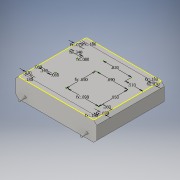
# Autodesk Inventor part: Chassis
Saved by Autodesk Inventor 2016 (Build 200138000, 138)
## iProperties
Created: 2015-09-02
Part Number: Chassis
Material: Generic
Document SubType Name: Modeling
Designer: lachesis
Density: 1 g/cm^3
Appearance: Default
Author: lachesis
Autodesk Inventor part; units mm, degrees
ref_plane "YZ Plane" through (0, 0, 0) normal (1, 0, 0) x (0, 1, 0)
ref_plane "XZ Plane" through (0, 0, 0) normal (0, 1, 0) x (-1, 0, 0)
ref_plane "XY Plane" through (0, 0, 0) normal (0, 0, 1) x (1, 0, 0)
sketch "Sketch1" plane through (0, 0, 0) normal (0, 0, 1) x (1, 0, 0)
  line L0 (-27.3831, 7.112) -> (27.3831, 7.112)
  line L1 (29.718, 4.7771) -> (29.718, -4.7771)
  line L2 (27.3831, -7.112) -> (-27.3831, -7.112)
  line L3 (-29.718, -4.7771) -> (-29.718, 4.7771)
  line L4 (-27.3831, 7.112) -> (-29.718, 4.7771)
  line L5 (-29.718, -4.7771) -> (-27.3831, -7.112)
  line L6 (27.3831, 7.112) -> (29.718, 4.7771)
  line L7 (29.718, -4.7771) -> (27.3831, -7.112)
  point P0 (0, 0)
  point P1 (-29.718, 7.112)
  point P2 (29.718, -7.112)
  point P3 (29.718, 7.112)
  point P4 (-29.718, -7.112)
  point P5 (29.718, 0)
  point P6 (0, 7.112)
  dimension "d0" = 59.436
  dimension "d1" = 14.224
  dimension "d4" = 3.302
  dimension "d5" = 135
  dimension "d7" = 45
  dimension "d8" = 3.302
  dimension "d10" = 45
  dimension "d11" = 3.302
  dimension "d13" = 45
  dimension "d14" = 3.302
  constraints: 16 end point, 8 point on line, 2 midpoint, 2 parallel, 1 horizontal, 1 horizontal alignment, 1 perpendicular, 1 vertical alignment
  measures "d0" distance between parallel lines of L1 L3
  measures "d1" distance between parallel lines of L0 L2
  measures "d4" distance of L0.start L3.end
  measures "d5" angle of L3 L4
  measures "d7" angle of L3 L5
  measures "d8" distance of L3.start L2.end
  measures "d10" angle of L0 L6
  measures "d11" distance of L0.end L1.start
  measures "d13" angle of L1 L7
  measures "d14" distance of L1.end L2.start
extrude "Extrusion1" add sketch "Sketch1" along normal blind 49.276
sketch "Sketch2" plane through (0, 0, 49.276) normal (0, 0, 1) x (1, 0, 0)
  circle A0 centre (-22.606, -3.556) radius 0.762
  line L0 (-27.3831, -7.112) -> (27.3831, -7.112) projected
  circle A1 centre (22.606, -3.556) radius 0.762
  line L1 (-29.718, 4.7771) -> (-29.718, -4.7771) projected
  line L2 (29.718, -4.7771) -> (29.718, 4.7771) projected
  point P0 (0, 0)
  dimension "d17" = 3.556
  dimension "d18" = 3.556
  dimension "d19" = 1.524
  dimension "d20" = 1.524
  dimension "d21" = 7.112
  dimension "d22" = 7.112
  constraints: 2 centre point
  measures "d17" distance from line of L0 A0.centre
  measures "d18" distance from line of L0 A1.centre
  measures "d19" diameter of A0
  measures "d20" diameter of A1
  measures "d21" distance from line of L1 A0.centre
  measures "d22" distance from line of L2 A1.centre
extrude "Extrusion2" add sketch "Sketch2" along normal blind 4.318
sketch "Sketch3" plane through (0, 0, 0) normal (0, 0, -1) x (-1, 0, 0)
  circle A0 centre (22.606, -3.556) radius 0.762 projected
  circle A1 centre (-22.606, -3.556) radius 0.762 projected
  circle A2 centre (-22.606, -3.556) radius 0.762
  circle A3 centre (22.606, -3.556) radius 0.762
  point P0 (0, 0)
  constraints: 2 centre point, 2 coincident, 2 concentric
extrude "Extrusion3" add sketch "Sketch3" along normal blind 4.318
sketch "Sketch4" plane through (-27.3831, 7.112, 0) normal (0, 1, 0) x (1, 0, 0)
  line L0 (0, 0) -> (0, -49.276) projected
  line L1 (54.7663, 0) -> (54.7663, -49.276) projected
  line L2 (0, -3.302) -> (54.7663, -3.302)
  line L3 (54.7663, -3.302) -> (54.7663, -45.974)
  line L4 (54.7663, -45.974) -> (0, -45.974)
  line L5 (0, -45.974) -> (0, -3.302)
  point P0 (27.3831, 0)
  dimension "d30" = 42.672
  dimension "d31" = 3.302
  constraints: 8 end point, 2 parallel, 2 point on line, 1 horizontal, 1 perpendicular
  measures "d30" distance between parallel lines of L4 L2
  measures "d31" distance from line of point (27.383, 0) L2
extrude "Extrusion4" cut sketch "Sketch4" against normal blind 11.8872
sketch "Sketch5" plane through (-27.3831, 7.112, 0) normal (0, 1, 0) x (1, 0, 0)
  line L0 (0, 0) -> (-2.3349, 0) projected
  line L1 (54.7663, -3.302) -> (54.7663, -45.974) projected
  line L2 (0, 0) -> (54.7663, 0)
  line L3 (54.7663, 0) -> (54.7663, -45.974)
  line L4 (54.7663, -45.974) -> (0, -45.974)
  line L5 (0, -45.974) -> (0, 0)
  point P0 (27.3831, 0)
  constraints: 8 end point, 2 parallel, 1 horizontal, 1 perpendicular
extrude "Extrusion5" add sketch "Sketch5" against normal blind 0.8128 separate body
sketch "Sketch6" plane through (-27.3831, 7.112, 0) normal (0, 1, 0) x (1, 0, 0)
  line L0 (0, -3.302) -> (0, -45.974) projected
  line L1 (54.7663, -3.302) -> (54.7663, -45.974) projected
  line L2 (54.7663, -49.276) -> (0, -49.276) projected
  line L3 (54.7663, 0) -> (0, 0) projected
  line L4 (0, 0) -> (0, -3.302) projected
  line L5 (0, -45.974) -> (0, -49.276) projected
  line L6 (54.7663, -45.974) -> (54.7663, -49.276) projected
  line L7 (54.7663, 0) -> (54.7663, -3.302) projected
  point P0 (27.3831, 0)
  point P1 (20.7303, -8.4836)
  point P2 (41.8123, -8.4836)
  point P3 (1.778, -4.572)
  point P4 (52.9883, -4.572)
  point P5 (1.778, -44.704)
  point P6 (52.9883, -44.704)
  point P7 (25.5563, -17.78)
  point P8 (48.1623, -17.78)
  point P9 (48.1623, -39.37)
  point P10 (25.5563, -39.37)
  point P11 (2.032, -35.052)
  point P12 (2.032, -14.224)
  point P13 (10.668, -33.02)
  point P14 (10.668, -16.256)
  dimension "d40" = 21.082
  dimension "d43" = 12.954
  dimension "d48" = 1.778
  dimension "d49" = 1.778
  dimension "d50" = 1.778
  dimension "d51" = 1.778
  dimension "d53" = 22.606
  dimension "d55" = 22.606
  dimension "d56" = 21.59
  dimension "d57" = 21.59
  dimension "d62" = 6.604
  dimension "d74" = 2.032
  dimension "d77" = 8.636
  dimension "d78" = 8.636
  dimension "d79" = 2.032
  dimension "d80" = 2.032
  dimension "d83" = 4.572
  dimension "d84" = 4.572
  dimension "d85" = 4.572
  dimension "d86" = 4.572
  constraints: 2 vertical alignment, 1 horizontal alignment
  measures "d40" distance of point (41.812, -8.484) point (20.73, -8.484)
  measures "d43" distance from line of L1 point (41.812, -8.484)
  measures "d48" distance from line of L0 point (1.778, -4.572)
  measures "d49" distance from line of L0 point (1.778, -44.704)
  measures "d50" distance from line of L1 point (52.988, -44.704)
  measures "d51" distance from line of L1 point (52.988, -4.572)
  measures "d53" distance of point (48.162, -17.78) point (25.556, -17.78)
  measures "d55" distance of point (48.162, -39.37) point (25.556, -39.37)
  measures "d56" distance of point (48.162, -39.37) point (48.162, -17.78)
  measures "d57" distance of point (25.556, -39.37) point (25.556, -17.78)
  measures "d62" distance from line of L1 point (48.162, -39.37)
  measures "d74" distance from line of L0 point (2.032, -35.052)
  measures "d77" horizontal distance of point (10.668, -33.02) point (2.032, -35.052)
  measures "d78" horizontal distance of point (2.032, -14.224) point (10.668, -16.256)
  measures "d79" vertical distance of point (10.668, -33.02) point (2.032, -35.052)
  measures "d80" vertical distance of point (10.668, -16.256) point (2.032, -14.224)
  measures "d83" distance from line of L2 point (1.778, -44.704)
  measures "d84" distance from line of L3 point (1.778, -4.572)
  measures "d85" distance from line of L2 point (52.988, -44.704)
  measures "d86" distance from line of L3 point (52.988, -4.572)
equation "\"d18\" = d17"
equation "\"d22\" = d21"
equation "\"d48\" = d49"
equation "\"d50\" = d48"
equation "\"d51\" = d48"
equation "\"d55\" = d53"
equation "\"d57\" = d56"
equation "\"d78\" = d77"
equation "\"d80\" = d79"
equation "\"d84\" = d83"
equation "\"d85\" = d83"
equation "\"d86\" = d83"
body "Solid1"
body "Solid2"
